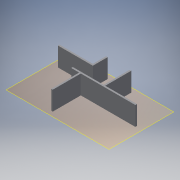
# Autodesk Inventor part: Wände_unten
Saved by Autodesk Inventor 2017 (Build 210142000, 142)
## iProperties
Created: 2017-06-01
Part Number: Wände_unten
Material: Generic
Document SubType Name: Modeling
Designer: Fake
Density: 1 g/cm^3
Appearance: Weiß
Author: Fake
Autodesk Inventor part; units mm, degrees
ref_plane "YZ Plane" through (0, 0, 0) normal (1, 0, 0) x (0, 1, 0)
ref_plane "XZ Plane" through (0, 0, 0) normal (0, 1, 0) x (-1, 0, 0)
ref_plane "XY Plane" through (0, 0, 0) normal (0, 0, 1) x (1, 0, 0)
ref_plane "Arbeitsebene1" through (0, 0, 1400) normal (0, 0, 1) x (1, 0, 0)
sketch "Skizze1" plane through (0, 0, 1400) normal (0, 0, 1) x (1, 0, 0)
  line L0 (5480, 3375) -> (5480, -3375) projected
  line L1 (5480, -3375) -> (-4000, -3375) projected
  line L2 (-4000, -3375) -> (-4000, -2075) projected
  line L3 (-4000, -2075) -> (-5480, -2075) projected
  line L4 (-5480, -2075) -> (-5480, 3375) projected
  line L5 (-5480, 3375) -> (5480, 3375) projected
  line L6 (-5480, -3575) -> (-5480, -2275) projected
  line L7 (-5480, -2275) -> (-4200, -2275) projected
  line L8 (-4200, -2275) -> (-4200, -3575) projected
  line L9 (-4200, -3575) -> (5680, -3575) projected
  line L10 (5680, -3575) -> (5680, 3575) projected
  line L11 (5680, 3575) -> (-5680, 3575) projected
  line L12 (-5680, 3575) -> (-5680, -3575) projected
  line L13 (-5680, -3575) -> (-5480, -3575) projected
  line L14 (-1140, -3375) -> (-1340, -3375)
  line L15 (-1340, -3375) -> (-1340, 25)
  line L16 (-1140, 25) -> (-1140, -3375)
  line L17 (-2310, 25) -> (-2310, 225)
  line L18 (5480, 225) -> (5480, 25)
  line L19 (-5480, 1775) -> (-1430, 1775)
  line L20 (-1230, 1575) -> (-5480, 1575)
  line L21 (-5480, 1575) -> (-5480, 1775)
  line L22 (-1230, 1575) -> (-1230, 3375)
  line L23 (-1430, 3375) -> (-1430, 1775)
  line L24 (1430, 3375) -> (1630, 3375)
  line L25 (1630, 3375) -> (1630, 225)
  line L26 (1430, 225) -> (1430, 3375)
  line L27 (5480, 25) -> (-1140, 25)
  line L28 (-1340, 25) -> (-2310, 25)
  line L29 (-2310, 225) -> (1430, 225)
  line L30 (1630, 225) -> (5480, 225)
  line L31 (-1430, 3375) -> (-1230, 3375)
  dimension "d0" = 6620
  dimension "d1" = 200
  dimension "d3" = 970
  dimension "d5" = 3850
  dimension "d6" = 3400
  dimension "d7" = 200
  dimension "d8" = 200
  dimension "d9" = 1600
  dimension "d10" = 200
  dimension "d11" = 200
  dimension "d12" = 4050
  constraints: 36 end point, 9 parallel, 5 horizontal, 5 point on line, 4 collinear, 4 perpendicular
  measures "d0" distance between parallel lines of L0 L16
  measures "d1" distance between parallel lines of L15 L16
  measures "d3" distance between parallel lines of L17 L15
  measures "d5" distance between parallel lines of L0 L25
  measures "d6" distance between parallel lines of L1 L27
  measures "d7" distance between parallel lines of L27 L29
  measures "d8" distance between parallel lines of L25 L26
  measures "d9" distance between parallel lines of L19 L5
  measures "d10" distance between parallel lines of L19 L20
  measures "d11" distance between parallel lines of L23 L22
  measures "d12" distance between parallel lines of L23 L4
ref_plane "Arbeitsebene2" through (-5680, -3575, 3700) normal (0, 0, 1) x (1, 0, 0)
extrude "Extrusion1" add sketch "Skizze1" along normal up to surface (2300 mm away) contours L0 L27 L16 L1 L15 L28 L17 L29 L26 L5 L25 L30 | L22 L20 L4 L19 L23 L5
sketch "Skizze2" plane through (-5480, 1575, 1400) normal (0, -1, 0) x (1, 0, 0)
  line L0 (4250, 2300) -> (0, 2300) projected
  line L1 (0, 0) -> (0, 2300) projected
  line L2 (0, 0) -> (4250, 0) projected
  line L3 (4250, 0) -> (4250, 2300) projected
  line L4 (4050, 0) -> (0, 0) projected
  line L5 (1700, 0) -> (2650, 0)
  line L6 (2650, 0) -> (2650, 1900)
  line L7 (2650, 1900) -> (1700, 1900)
  line L8 (1700, 1900) -> (1700, 0)
  dimension "d15" = 950
  dimension "d16" = 1600
  dimension "d17" = 1900
  constraints: 8 end point, 2 parallel, 1 horizontal, 1 perpendicular, 1 point on line
  measures "d15" distance of L6.end L7.end
  measures "d16" distance between parallel lines of L6 L3
  measures "d17" distance of L7.end L5.start
extrude "Extrusion2" cut sketch "Skizze2" against normal blind 879.25 contours L8 L7 L6 L2
sketch "Skizze3" plane through (1430, 225, 1400) normal (-1, 0, 0) x (0, 0, 1)
  line L0 (2300, 0) -> (2300, 3150) projected
  line L1 (0, 3150) -> (2300, 3150) projected
  line L2 (0, 3150) -> (0, 0) projected
  line L3 (0, 0) -> (2300, 0) projected
  line L4 (0, 1750) -> (1900, 1750)
  line L5 (1900, 1750) -> (1900, 800)
  line L6 (1900, 800) -> (0, 800)
  line L7 (0, 800) -> (0, 1750)
  dimension "d20" = 1900
  dimension "d21" = 950
  dimension "d22" = 1400
  constraints: 8 end point, 2 parallel, 1 horizontal, 1 perpendicular, 1 point on line
  measures "d20" distance between parallel lines of L2 L5
  measures "d21" distance between parallel lines of L6 L4
  measures "d22" distance between parallel lines of L1 L4
extrude "Extrusion3" cut sketch "Skizze3" against normal blind 879.25 contours L2 L4 L5 L6
sketch "Skizze4" plane through (-2310, 225, 1400) normal (0, 1, 0) x (1, 0, 0)
  line L0 (0, -2300) -> (3740, -2300) projected
  line L1 (3740, 0) -> (3740, -2300) projected
  line L2 (3740, 0) -> (0, 0) projected
  line L3 (0, 0) -> (0, -2300) projected
  line L4 (3740, 0) -> (0, 0) projected
  line L5 (2310, 0) -> (1360, 0)
  line L6 (1360, 0) -> (1360, -1900)
  line L7 (1360, -1900) -> (2310, -1900)
  line L8 (2310, -1900) -> (2310, 0)
  dimension "d25" = 1900
  dimension "d26" = 950
  dimension "d27" = 1360
  constraints: 8 end point, 2 parallel, 1 horizontal, 1 perpendicular, 1 point on line
  measures "d25" distance between parallel lines of L2 L7
  measures "d26" distance between parallel lines of L6 L8
  measures "d27" distance between parallel lines of L6 L3
extrude "Extrusion4" cut sketch "Skizze4" against normal blind 879.25 contours L2 L8 L7 L6
